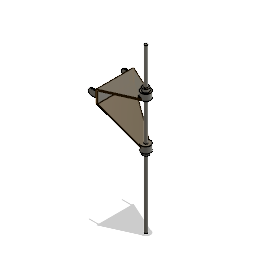
Strider v1 v3 (Autodesk Fusion 360 design; units mm, degrees)
Autodesk Fusion 360 part; units mm, degrees
note: some values were not read from the file. Chosen so that the rebuilt part matches the saved one: which pieces of a blend or face edit are solid. Set by a fixed rule: which sketch regions a step uses.
sketch "Sketch1" plane through (0, 0, 0) normal (0, 1, 0) x (1, 0, 0)
  circle A0 centre (0, 0) radius 19.05
  circle A1 centre (0, 0) radius 6.35
  line L0 (-126.6752, -0.283) -> (-126.6752, 76.5245)
  line L1 (-126.6752, 76.5245) -> (-126.6752, -75.8755)
  line L2 (0, 19.05) -> (-126.6752, 76.5245)
  line L3 (0, -19.05) -> (-126.6752, -75.8755)
  dimension "d1" = 38.1
  dimension "d3" = 12.7
  dimension "d4" = 152.4
  measures "d1" diameter of A0
  measures "d3" diameter of A1
extrude "Extrude1" add sketch "Sketch1" along normal blind 4.7625 contours A0 L0 L1 L2 L3 makes body 1
sketch "Sketch2" plane through (0, 0, 0) normal (0, 1, 0) x (1, 0, 0)
  circle A0 centre (0, 0) radius 19.05
  dimension "d7" = 38.1
  measures "d7" diameter of A0
extrude "Extrude2" add sketch "Sketch2" along normal blind 25.4 bodies 1
sketch "Sketch3" plane through (0, 25.4, 0) normal (0, 1, 0) x (-1, 0, 0)
  circle A0 centre (0, 0) radius 19.05
  circle A1 centre (0, 0) radius 12.7
  dimension "d10" = 25.4
  measures "d10" diameter of A1
extrude "Extrude3" add sketch "Sketch3" along normal blind 12.7 contours A1 bodies 1
sketch "Sketch4" plane through (0, 38.1, 0) normal (0, 1, 0) x (-1, 0, 0)
  circle A0 centre (0, 0) radius 12.7
  circle A1 centre (0, 0) radius 6.35
  dimension "d13" = 12.7
  measures "d13" diameter of A1
extrude "Extrude4" cut sketch "Sketch4" against normal up to surface (38.1 mm away) contours A1 bodies 1
fillet "Fillet1" radius 2.54 1 edges at (-19.05, 4.7625, 0) on bodies 1
sketch "Sketch5" plane through (-126.6752, 0, 0) normal (-1, 0, 0) x (0, 0, 1)
  line L0 (-76.5245, 0) -> (75.8755, 0)
  line L1 (75.8755, 0) -> (75.8755, 4.7625)
  line L2 (75.8755, 4.7625) -> (-76.5245, 4.7625)
  line L3 (-76.5245, 4.7625) -> (-76.5245, 0)
  line L4 (-76.5245, 4.7625) -> (75.8755, 4.7625)
  line L5 (-76.5245, 4.7625) -> (75.8755, 4.7625)
  line L6 (75.8755, 4.7625) -> (75.8755, -46.0375)
  line L7 (75.8755, -46.0375) -> (-76.5245, -46.0375)
  line L8 (-76.5245, -46.0375) -> (-76.5245, 4.7625)
  dimension "d17" = 50.8
  measures "d17" distance of origin
extrude "Extrude5" add sketch "Sketch5" against normal blind 4.7625 contours L0 L6 L7 L8 bodies 1
move_face "OffsetFaces1" offset -46.99 1 faces at (-123.5002, 0, 75.1633) on bodies 1
move_face "OffsetFaces2" offset -46.99 1 faces at (-123.5002, 0, -75.8043) on bodies 1
fillet "Fillet2" radius 2.54 1 edges at (-121.9127, 0, -0.3123) on bodies 1
sketch "Sketch6" plane through (-126.6752, 0, 0) normal (-1, 0, 0) x (0, 0, 1)
  line L0 (-76.5245, 4.7625) -> (-76.5245, -46.0375)
  line L1 (-76.5245, -46.0375) -> (75.8755, -46.0375)
  line L2 (75.8755, -46.0375) -> (75.8755, 4.7625) construction
  line L3 (75.8755, 4.7625) -> (-76.5245, 4.7625)
  line L4 (69.6875, -7.8625) -> (64.925, -7.8625)
  line L5 (64.925, -7.8625) -> (64.925, -33.2625)
  line L6 (64.925, -33.2625) -> (69.6875, -33.2625)
  line L7 (69.6875, -33.2625) -> (69.6875, -7.8625)
  dimension "d27" = 4.7625
  dimension "d28" = 25.4
  dimension "d29" = 4.7625
  measures "d28" distance of origin
extrude "Extrude6" add sketch "Sketch6" along normal blind 38.1 bodies 1
sketch "Sketch7" plane through (0, 0, 64.925) normal (0, 0, -1) x (-1, 0, 0)
  line L0 (126.6752, -7.8625) -> (126.6752, -33.2625)
  line L1 (126.6752, -33.2625) -> (164.7752, -33.2625)
  line L2 (164.7752, -33.2625) -> (164.7752, -7.8625)
  line L3 (164.7752, -7.8625) -> (126.6752, -7.8625)
  circle A0 centre (152.0752, -20.5625) radius 12.7
extrude "Extrude7" add sketch "Sketch7" along normal blind -2.54 and the other way blind 0 contours A0 bodies 1
sketch "Sketch8" plane through (0, 0, 64.925) normal (0, 0, -1) x (-1, 0, 0)
  line L0 (126.6752, -33.2625) -> (164.7752, -33.2625)
  line L1 (164.7752, -33.2625) -> (164.7752, -7.8625)
  line L2 (164.7752, -7.8625) -> (126.6752, -7.8625)
  line L3 (126.6752, -7.8625) -> (126.6752, -33.2625)
  circle A0 centre (152.0752, -20.5625) radius 12.7
  circle A1 centre (152.0752, -20.5625) radius 12.7
extrude "Extrude8" cut sketch "Sketch8" along normal blind 4.7625 from surface at -4.7625 contours A0 A1 bodies 1
delete_face "DeleteFace1" 1 faces at (-162.2801, -30.7674, 64.925) on bodies 1
delete_face "DeleteFace2" 1 faces at (-162.2801, -10.3575, 64.925) on bodies 1
extrude "Extrude9" add sketch "Sketch8" against normal blind 4.7625 contours A0 A1 bodies 1
fillet "Fillet3" radius 2.54 1 edges at (-126.6752, -20.5625, 64.925) on bodies 1
fillet "Fillet4" radius 2.54 1 edges at (-126.6752, -33.2625, 66.0363) on bodies 1
fillet "Fillet5" radius 2.54 1 edges at (-126.6752, -21.8325, 69.6875) on bodies 1
fillet "Fillet6" radius 2.54 1 edges at (-126.6752, -7.8625, 67.3063) on bodies 1
mirror "Mirror1" about plane through (0, 0, 0) normal (0, 0, 1) of 9 faces at (-126.6957, -16.3291, 62.7073) (-144.4552, -33.2625, 66.5125) (-126.6803, -25.4819, 72.066) (-126.6803, -5.4839, 68.7861) (-144.4552, -24.7958, 69.6875) (-136.8352, -7.8625, 68.1) (-126.6803, -35.641, 65.8265) (-159.7435, -30.686, 68.1) (-144.4552, -24.7958, 64.925) on bodies 1
sketch "Sketch9" plane through (7.1141, 0, 15.8587) normal (0.409296, 0, 0.912402) x (0.912402, 0, -0.409296)
  line L0 (-146.6342, -46.0375) -> (-141.4144, -46.0375)
  line L1 (-141.4144, -46.0375) -> (-141.4144, -2.54)
  ellipse E0 centre (-138.6306, -2.54) end of major axis (-141.4144, -2.54) minor radius 2.54 (-138.6306, 0) -> (-141.4144, -2.54) ccw
  line L2 (-138.6306, 0) -> (-7.7971, 0)
  line L3 (-7.7971, 0) -> (-7.7971, 7.3025)
  spline S0 degree 3 poles (-12.807, 4.7625) (-12.1585, 4.7625) (-11.3875, 4.8694) (-10.1868, 5.1894) (-9.5221, 5.4469) (-8.6636, 5.9593) (-8.277, 6.255) (-7.9698, 6.6949) (-7.8957, 6.8335) (-7.8196, 7.0622) (-7.7971, 7.1924) (-7.7971, 7.3025) knots 0.487 0.487 0.487 0.487 0.681573 0.681573 0.859792 0.859792 0.981491 0.981491 1.020768 1.020768 1.0538 1.0538 1.0538 1.0538
  line L4 (-12.807, 4.7625) -> (-146.6342, 4.7625)
  line L5 (-146.6342, 4.7625) -> (-146.6342, -46.0375)
sketch "Sketch10" plane through (0, 0, 0) normal (1, 0, 0) x (0, 0, -1)
sketch "Sketch11" plane through (0, 0, 0) normal (1, 0, 0) x (0, 0, -1)
sketch "Sketch12" plane through (-126.6752, 0, 0) normal (-1, 0, 0) x (0, 0, 1)
  line L0 (-62.385, -35.8025) -> (-72.2275, -35.8025)
  line L1 (-72.2275, -35.8025) -> (-72.2275, -5.3225)
  line L2 (-72.2275, -5.3225) -> (-62.385, -5.3225)
  line L3 (-62.385, -5.3225) -> (-62.385, -35.8025)
  line L4 (-76.5245, 4.7625) -> (-76.5245, -46.0375)
  line L5 (-76.5245, -46.0375) -> (75.8755, -46.0375)
  line L6 (75.8755, -46.0375) -> (75.8755, 4.7625)
  line L7 (75.8755, 4.7625) -> (-76.5245, 4.7625)
  line L8 (72.2275, -35.8025) -> (62.385, -35.8025)
  line L9 (62.385, -35.8025) -> (62.385, -5.3225)
  line L10 (62.385, -5.3225) -> (72.2275, -5.3225)
  line L11 (72.2275, -5.3225) -> (72.2275, -35.8025)
ref_plane "WorkPlane1" through (0, -158.75, 0) normal (0, 1, 0) x (0, 0, 1)
sketch "Sketch13" plane through (0, -158.75, 0) normal (0, 1, 0) x (1, 0, 0)
  circle A0 centre (0, 0) radius 19.05
  dimension "d51" = 38.1
  measures "d51" diameter of A0
ref_plane "WorkPlane2" through (-121.9127, -46.0375, -0.3123) normal (0.707107, 0.707107, 0) x (0, 0, -1)
sketch "Sketch14" plane through (-121.9127, -46.0375, -0.3123) normal (0.707107, 0.707107, 0) x (0, 0, -1)
ref_plane "WorkPlane3" through (-121.9127, -46.0375, -0.3123) normal (0.707107, 0.707107, 0) x (0, 0, -1)
sketch "Sketch15" plane through (-121.9127, -46.0375, -0.3123) normal (0.707107, 0.707107, 0) x (0, 0, -1)
  line L0 (-74.0514, 0) -> (-19.3527, -165.4768)
  line L1 (74.0514, 0) -> (18.7266, -165.4459)
  line L2 (-74.0514, 0) -> (74.0514, 0)
  line L3 (18.7266, -165.4459) -> (15.5882, -174.8312)
  line L4 (-19.3527, -165.4768) -> (-16.2468, -174.8729)
  line L5 (-16.2468, -174.8729) -> (15.5882, -174.8312)
extrude "Extrude10" add sketch "Sketch13" against normal blind 25.4 separate body makes body 2
sketch "Sketch16" plane through (0, -184.15, 0) normal (0, -1, 0) x (1, 0, 0)
  circle A0 centre (0, 0) radius 19.05
  circle A1 centre (0, 0) radius 12.7
  dimension "d56" = 25.4
  measures "d56" diameter of A1
extrude "Extrude11" add sketch "Sketch16" along normal blind 12.7 contours A1 bodies 2
sketch "Sketch17" plane through (0, -158.75, 0) normal (0, 1, 0) x (-1, 0, 0)
  circle A0 centre (0, 0) radius 19.05
  circle A1 centre (0, 0) radius 6.35
extrude "Extrude12" cut sketch "Sketch17" against normal up to surface (38.1 mm away) contours A1 bodies 2
extrude "Extrude13" add sketch "Sketch15" against normal blind 4.7625 separate body makes body 3
sketch "Sketch18" plane through (7.1677, 0, -15.7979) normal (0.413177, 0, -0.910651) x (-0.910651, 0, -0.413177)
  line L0 (141.7453, -46.0375) -> (146.975, -46.0375)
  line L1 (146.975, -46.0375) -> (146.975, 4.7625)
  line L2 (146.975, 4.7625) -> (12.8522, 4.7625)
  spline S0 degree 3 poles (7.871, 7.3025) (7.871, 7.192) (7.8935, 7.0613) (7.9694, 6.8319) (8.0432, 6.693) (8.3485, 6.2533) (8.7328, 5.9573) (9.5856, 5.4456) (10.2458, 5.1886) (11.4396, 4.8691) (12.2068, 4.7625) (12.8522, 4.7625) knots 1.050606 1.050606 1.050606 1.050606 1.08376 1.08376 1.123088 1.123088 1.244351 1.244351 1.421468 1.421468 1.615092 1.615092 1.615092 1.615092
  line L3 (7.871, 7.3025) -> (7.871, 0)
  line L4 (7.871, 0) -> (138.956, 0)
  ellipse E0 centre (138.956, -2.54) end of major axis (141.7453, -2.54) minor radius 2.54 (141.7453, -2.54) -> (138.956, 0) ccw
  line L5 (141.7453, -2.54) -> (141.7453, -46.0375)
sketch "Sketch19" plane through (0, 0, 0) normal (0, 0, 1) x (1, 0, 0)
sketch "Sketch20" plane through (-63.3376, -19.3675, -47.7873) normal (0.413177, 0, -0.910651) x (-0.910651, 0, -0.413177)
loft "Loft1" add section 1 face at (-124.1578, -48.2826, 24.3715) section 2 face at (-125.0877, -46.0375, -25.0043) on bodies 1 3 bodies 3 1
sketch "Sketch21" plane through (-83.9751, -83.9751, 0) normal (0.707107, 0.707107, 0) x (0, 0, -1)
  line L0 (-73.739, 53.6519) -> (-15.9345, -121.2211)
  line L1 (-15.9345, -121.2211) -> (15.9005, -121.1793)
  line L2 (15.9005, -121.1793) -> (74.3637, 53.6519)
  line L3 (74.3637, 53.6519) -> (-73.739, 53.6519)
sketch "Sketch22" plane through (0, -158.75, 0) normal (0, 1, 0) x (-1, 0, 0)
  circle A0 centre (0, 0) radius 6.35
  circle A1 centre (0, 0) radius 19.05
extrude "Extrude14" cut sketch "Sketch22" against normal up to surface (38.1 mm away) contours A0 bodies 3
ref_plane "WorkPlane1" through (0, 187.325, 0) normal (0, 1, 0) x (0, 0, 1) in component "Component"
sketch "Sketch1 (2)" plane through (0, 187.325, 0) normal (0, 1, 0) x (1, 0, 0) in component "Component"
  circle A0 centre (0, 0) radius 6.35
extrude "Extrude1'" add sketch "Sketch1 (2)" against normal blind 660.4 separate body makes body 4 in component "Component"
component "Component" placed x (1, 0, 0) y (0, 1, 0) z (0, 0, 1) at (0, 0, 0)
equation "d5 = ( 3 / 16 ) * 1 in"
equation "d19 = ( -3 / 16 ) * 1 in"
equation "d27 = ( 3 / 16 ) * 1 in"
equation "d29 = ( 3 / 16 ) * 1 in"
equation "d41 = ( 3 / 16 ) * 1 in"
equation "d43 = ( -3 / 16 ) * 1 in"
equation "d50 = -6 1/4\""
equation "d61 = ( -3 / 16 ) * 1 in"
equation "d65 = 7 3/8\""
